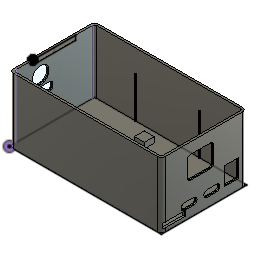
server_spiers_box v25 (Autodesk Fusion 360 design; units mm, degrees)
Autodesk Fusion 360 part; units mm, degrees
sketch "Base" plane through (0, 0, 0) normal (0, 1, 0) x (1, 0, 0) in component "Case"
  line L0 (0, 0) -> (107, 0)
  line L1 (107, 0) -> (107, 60)
  line L2 (107, 60) -> (0, 60)
  line L3 (0, 60) -> (0, 0)
  dimension "d6" = 107
  dimension "d7" = 60
  constraint horizontal L0
  constraint vertical L1
  constraint horizontal L2
  constraint vertical L3
  constraint coincident L0.start L3.end
  measures "d6" distance of L0.start L0.end
  measures "d7" distance of L0.start L2.end
extrude "Extrude1" add sketch "Base" along normal blind 46 makes body 1 in component "Case"
fillet "Fillet1" radius 3 4 edges at (107, 23, 0) (0, 23, 0) (107, 23, -60) (0, 23, -60) on bodies 1 in component "Case"
shell "Shell1" thickness 1.5 removed faces 1 at (36.6667, 46, -40) on bodies 1 in component "Case"
sketch "Knob" plane through (1.5, 0, 0) normal (1, 0, 0) x (0, 0, -1) in component "Case"
  line L0 (57, 46) -> (3, 46)
  line L1 (3, 1.5) -> (57, 1.5)
  line L2 (15, 46) -> (45, 46)
  line L3 (45, 46) -> (45, 43)
  line L4 (45, 43) -> (15, 43)
  line L5 (15, 43) -> (15, 46)
  line L6 (30, 46) -> (30, 43) construction
  line L7 (57, 1.5) -> (57, 46)
  line L8 (3, 46) -> (3, 1.5)
  dimension "d12" = 30
  dimension "d13" = 3
  constraint horizontal L2
  constraint vertical L3
  constraint horizontal L4
  constraint vertical L5
  constraint coincident L0 L2.start
  constraint midpoint L0 L6.start
  constraint midpoint L4 L6.end
  constraint vertical L6
  measures "d12" distance of L3.end L4.end
  measures "d13" distance of L2.end L3.end
extrude "Extrude2" add sketch "Knob" along normal blind 6 draft -45 contours L0 L2 L3 L4 L5 bodies 1 in component "Case"
ref_plane "WorkPlane2" through (53.5, 23, -30) normal (-1, 0, 0) x (0, 0, 1) in component "Case"
mirror "Mirror1" about plane through (53.5, 23, -30) normal (-1, 0, 0) of "Extrude2" in component "Case"
sketch "Top" plane through (0, 46, 0) normal (0, 1, 0) x (-1, 0, 0) in component "Top Cover"
  line L0 (-107, -3) -> (-107, -57)
  arc A0 (-107, -57) -> (-104, -60) centre (-104, -57) ccw
  line L1 (-104, -60) -> (-3, -60)
  arc A1 (-3, -60) -> (0, -57) centre (-3, -57) ccw
  line L2 (0, -57) -> (0, -3)
  arc A2 (0, -3) -> (-3, 0) centre (-3, -3) ccw
  line L3 (-3, 0) -> (-104, 0)
  arc A3 (-104, 0) -> (-107, -3) centre (-104, -3) ccw
  line L4 (-105.5, -15) -> (-105.5, -3)
  line L5 (-104, -1.5) -> (-3, -1.5)
  line L6 (-1.5, -3) -> (-1.5, -15)
  line L7 (-1.5, -15) -> (-1.5, -45)
  line L8 (-1.5, -45) -> (-1.5, -57)
  line L9 (-3, -58.5) -> (-104, -58.5)
  line L10 (-105.5, -45) -> (-105.5, -15)
  arc A4 (-104, -1.5) -> (-105.5, -3) centre (-104, -3) ccw
  arc A5 (-1.5, -3) -> (-3, -1.5) centre (-3, -3) ccw
  arc A6 (-3, -58.5) -> (-1.5, -57) centre (-3, -57) ccw
  arc A7 (-105.5, -57) -> (-104, -58.5) centre (-104, -57) ccw
  line L11 (-105.5, -57) -> (-105.5, -45)
extrude "Extrude1'" add sketch "Top" along normal blind 1.5 separate body contours L0 A0 L1 A1 L2 A2 L3 A3 | L4 L5 L6 L7 L8 L9 L10 A4 A5 A6 A7 L11 makes body 2 in component "Top Cover"
sketch "Lip" plane through (0, 46, 0) normal (0, -1, 0) x (1, 0, 0) in component "Top Cover"
  arc A0 (107, -3) -> (104, 0) centre (104, -3) ccw
  line L0 (104, 0) -> (3, 0)
  arc A1 (3, 0) -> (0, -3) centre (3, -3) ccw
  line L1 (0, -3) -> (0, -57)
  arc A2 (0, -57) -> (3, -60) centre (3, -57) ccw
  line L2 (3, -60) -> (104, -60)
  arc A3 (104, -60) -> (107, -57) centre (104, -57) ccw
  line L3 (107, -57) -> (107, -3)
  line L4 (107, -3) -> (107, -57)
  line L5 (105.3, -57) -> (105.3, -3)
  arc A4 (105.3, -3) -> (104, -1.7) centre (104, -3) ccw
  line L6 (104, -1.7) -> (3, -1.7)
  arc A5 (3, -1.7) -> (1.7, -3) centre (3, -3) ccw
  line L7 (1.7, -3) -> (1.7, -57)
  arc A6 (1.7, -57) -> (3, -58.3) centre (3, -57) ccw
  line L8 (3, -58.3) -> (104, -58.3)
  arc A7 (104, -58.3) -> (105.3, -57) centre (104, -57) ccw
  dimension "d19" = 1.7
  dimension "d31" = 1.7
  measures "d31" distance of L4 L5
extrude "Extrude2'" add sketch "Lip" along normal blind 3 contours L5 A4 L6 A5 L7 A6 L8 A7 bodies 2 in component "Top Cover"
extrude "Extrude3" cut sketch "Knob" along normal blind 3 draft -45 from surface at 0.2 contours L0 L2 L3 L4 L5 bodies 2 in component "Top Cover"
ref_plane "WorkPlane2" through (53.5, 0, 0) normal (1, 0, 0) x (0, 1, 0) in component "Top Cover"
mirror "Mirror1'" about plane through (53.5, 0, 0) normal (1, 0, 0) of "Extrude3" in component "Top Cover"
shell "Shell1'" thickness 1.5 removed faces 1 at (36.2333, 43, -25) on bodies 2 in component "Top Cover"
chamfer "Chamfer1" distance 0.6 angle 45 2 edges at (1.7, 43, -30) (105.3, 43, -30) on bodies 2 in component "Top Cover"
sketch "Esquisse1" plane through (107, 0, 0) normal (1, 0, 0) x (0, 0, -1)
  line L0 (57, 46) -> (3, 46)
  line L1 (3, 46) -> (3, 0)
  line L2 (3, 0) -> (57, 0)
  line L3 (57, 0) -> (57, 46)
  line L4 (38.75, 10.7) -> (32.25, 10.7)
  line L5 (32.25, 10.7) -> (32.25, 6.7)
  line L6 (32.25, 6.7) -> (38.75, 6.7)
  line L7 (38.75, 6.7) -> (38.75, 10.7)
  line L8 (38.75, 10.7) -> (32.25, 6.7) construction
  line L9 (32.25, 10.7) -> (38.75, 6.7) construction
  line L10 (60, 0) -> (60, 46)
  line L11 (0, 0) -> (60, 0)
  line L12 (22.75, 10.7) -> (16.25, 10.7)
  line L13 (16.25, 10.7) -> (16.25, 6.7)
  line L14 (16.25, 6.7) -> (22.75, 6.7)
  line L15 (22.75, 6.7) -> (22.75, 10.7)
  line L16 (22.75, 10.7) -> (16.25, 6.7) construction
  line L17 (16.25, 10.7) -> (22.75, 6.7) construction
  circle A0 centre (38.75, 8.7) radius 2
  circle A1 centre (32.25, 8.7) radius 2
  circle A2 centre (22.75, 8.7) radius 2
  circle A3 centre (16.25, 8.7) radius 2
  line L18 (34.5, 38) -> (20.5, 38)
  line L19 (18.5, 36) -> (18.5, 25)
  line L20 (20.5, 23) -> (34.5, 23)
  line L21 (36.5, 25) -> (36.5, 36)
  line L22 (36.5, 38) -> (18.5, 23) construction
  line L23 (18.5, 38) -> (36.5, 23) construction
  arc A4 (20.5, 38) -> (18.5, 36) centre (20.5, 36) ccw
  arc A5 (36.5, 36) -> (34.5, 38) centre (34.5, 36) ccw
  arc A6 (34.5, 23) -> (36.5, 25) centre (34.5, 25) ccw
  arc A7 (18.5, 25) -> (20.5, 23) centre (20.5, 25) ccw
  line L24 (54.25, 7.2) -> (44.75, 7.2)
  line L25 (44.75, 7.2) -> (44.75, 19.2)
  line L26 (44.75, 19.2) -> (54.25, 19.2)
  line L27 (54.25, 19.2) -> (54.25, 7.2)
  line L28 (54.25, 7.2) -> (44.75, 19.2) construction
  line L29 (44.75, 7.2) -> (54.25, 19.2) construction
  line L30 (0, 46) -> (0, 0)
  line L31 (16.5, 2.5) -> (1.5, 2.5)
  line L32 (1.5, 2.5) -> (1.5, 5.7)
  line L33 (1.5, 5.7) -> (16.5, 5.7)
  line L34 (16.5, 5.7) -> (16.5, 2.5)
  line L35 (16.5, 2.5) -> (1.5, 5.7) construction
  line L36 (1.5, 2.5) -> (16.5, 5.7) construction
  point P0 (35.5, 8.7)
  point P1 (19.5, 8.7)
  point P2 (27.5, 30.5)
  point P3 (49.5, 13.2)
  point P4 (9, 4.1)
  dimension "d36" = 6.5
  dimension "d37" = 4
  dimension "d39" = 8.7
  dimension "d40" = 6.5
  dimension "d41" = 4
  dimension "d42" = 16
  dimension "d43" = 8.7
  dimension "d44" = 4
  dimension "d45" = 4
  dimension "d46" = 4
  dimension "d47" = 4
  dimension "d69" = 18
  dimension "d70" = 15
  dimension "d71" = 30.5
  dimension "d72" = 32.5
  dimension "d82" = 2
  dimension "d83" = 2
  dimension "d84" = 2
  dimension "d85" = 2
  dimension "d233" = 9.5
  dimension "d234" = 12
  dimension "d235" = 13.2
  dimension "d236" = 10.5
  dimension "d237" = 14
  dimension "d260" = 15
  dimension "d261" = 3.2
  dimension "d262" = 9
  dimension "d335" = 4.6
  constraint horizontal L4
  constraint perpendicular L4 L5
  constraint parallel L4 L6
  constraint parallel L5 L7
  constraint coincident L8 P0
  constraint coincident L9 P0
  constraint horizontal L12
  constraint perpendicular L12 L13
  constraint parallel L12 L14
  constraint parallel L13 L15
  constraint coincident L16 P1
  constraint coincident L17 P1
  constraint coincident L4.start A0
  constraint midpoint L7 A0.centre
  constraint midpoint L5 A1.centre
  constraint midpoint L15 A2.centre
  constraint midpoint L13 A3.centre
  constraint horizontal L18
  constraint perpendicular L18 L19
  constraint parallel L18 L20
  constraint parallel L19 L21
  constraint coincident L22 P2
  constraint coincident L23 P2
  constraint coincident L23.start L18
  constraint coincident L23.start L19
  constraint tangent L18 A4
  constraint tangent L19 A4
  constraint coincident L22.start L18
  constraint coincident L22.start L21
  constraint tangent L18 A5
  constraint tangent L21 A5
  constraint coincident L23.end L20
  constraint coincident L23.end L21
  constraint tangent L20 A6
  constraint tangent L21 A6
  constraint coincident L22.end L19
  constraint coincident L22.end L20
  constraint tangent L19 A7
  constraint tangent L20 A7
  constraint horizontal L24
  constraint perpendicular L24 L25
  constraint parallel L24 L26
  constraint parallel L25 L27
  constraint coincident L28 P3
  constraint coincident L29 P3
  constraint horizontal L31
  constraint perpendicular L31 L32
  constraint parallel L31 L33
  constraint parallel L32 L34
  constraint coincident L35 P4
  constraint coincident L36 P4
  measures "d36" distance of L5.end L6.end
  measures "d37" distance of L4.end L5.end
  measures "d39" distance of P0 L11
  measures "d40" distance of L13.end L14.end
  measures "d41" distance of L12.end L13.end
  measures "d42" horizontal distance of P0 P1
  measures "d43" distance of L11 P1
  measures "d44" diameter of A0
  measures "d45" diameter of A1
  measures "d46" diameter of A2
  measures "d47" diameter of A3
  measures "d69" distance of L22.end L23.end
  measures "d70" distance of L23.start L22.end
  measures "d71" distance of L11 P2
  measures "d72" distance of L10 P2
  measures "d82" radius of A4
  measures "d83" radius of A5
  measures "d84" radius of A6
  measures "d85" radius of A7
  measures "d233" distance of L25.end L26.end
  measures "d234" distance of L24.end L25.end
  measures "d235" distance of L11 P3
  measures "d236" distance of L10 P3
  measures "d237" horizontal distance of P0 P3
  measures "d260" distance of L32.end L33.end
  measures "d261" distance of L31.end L32.end
  measures "d262" distance of L30 P4
  measures "d335" vertical distance of A3.centre P4
extrude "Extrusion3" cut sketch "Esquisse1" against normal blind 1.5 contours L4 L6 A0 A1 | L7 A0 | L7 A0 | L5 A1 | L5 A1 bodies 1 in component "Case"
extrude "Extrusion1" [suppressed]
extrude "Extrusion4" cut sketch "Esquisse1" against normal blind 1.5 contours L12 L14 A2 A3 | L15 A2 | L15 A2 | L13 A3 | L13 A3 bodies 1 in component "Case"
extrude "Extrusion9" cut sketch "Esquisse1" against normal blind 1.5 contours L18 L19 L20 L21 A4 A5 A6 A7 bodies 1 in component "Case"
fillet "Congé27" radius 0.375 8 edges at (105.5, 30.5, -18.5) (105.5, 23.5858, -19.0858) (105.5, 23, -27.5) (105.5, 23.5858, -35.9142) (105.5, 30.5, -36.5) (105.5, 37.4142, -35.9142) (105.5, 38, -27.5) (105.5, 37.4142, -19.0858) on bodies 1 in component "Case"
fillet "Congé28" radius 0.375 4 edges at (105.5, 6.7, -35.5) (105.5, 8.7, -40.75) (105.5, 10.7, -35.5) (105.5, 8.7, -30.25) on bodies 1 in component "Case"
fillet "Congé29" radius 0.375 4 edges at (105.5, 6.7, -19.5) (105.5, 8.7, -24.75) (105.5, 10.7, -19.5) (105.5, 8.7, -14.25) on bodies 1 in component "Case"
fillet "Congé30" radius 0.375 8 edges at (107, 30.5, -18.5) (107, 37.4142, -19.0858) (107, 38, -27.5) (107, 37.4142, -35.9142) (107, 30.5, -36.5) (107, 23.5858, -35.9142) (107, 23, -27.5) (107, 23.5858, -19.0858) on bodies 1 in component "Case"
fillet "Congé32" radius 0.375 4 edges at (107, 10.7, -19.5) (107, 8.7, -24.75) (107, 6.7, -19.5) (107, 8.7, -14.25) on bodies 1 in component "Case"
fillet "Congé33" radius 0.375 4 edges at (107, 10.7, -35.5) (107, 8.7, -40.75) (107, 6.7, -35.5) (107, 8.7, -30.25) on bodies 1 in component "Case"
extrude "Extrusion22" cut sketch "Esquisse1" against normal blind 1.5 contours L24 L25 L26 L27 bodies 1 in component "Case"
chamfer "Chanfrein6" distance 0.75 angle 45 1 edges at (105.5, 19.2, -49.5) on bodies 1 in component "Case"
fillet "Congé40" radius 0.375 3 edges at (105.5, 13.575, -44.75) (105.5, 7.2, -49.5) (105.5, 13.575, -54.25) on bodies 1 in component "Case"
fillet "Congé41" radius 0.375 4 edges at (107, 7.2, -49.5) (107, 13.2, -54.25) (107, 13.2, -44.75) (107, 19.2, -49.5) on bodies 1 in component "Case"
extrude "Extrusion29" cut sketch "Esquisse1" against normal blind 2.5 contours L1 L31 L33 L34 | L1 L31 L32 L33 bodies 1 in component "Case"
chamfer "Chanfrein9" distance 0.75 angle 45 2 edges at (105.5, 5.7, -9.75) (105.2247, 5.7, -2.134) on bodies 1 in component "Case"
fillet "Congé49" radius 0.375 1 edges at (107, 4.1, -16.5) on bodies 1 in component "Case"
fillet "Congé50" radius 0.375 2 edges at (106.8978, 5.7, -2.2235) (107, 5.7, -9.9375) on bodies 1 in component "Case"
sketch "Esquisse2" plane through (0, -0.0808, 0.0705) normal (-1, 0, 0) x (0, 0, 1)
  line L0 (-57.0705, 46.0808) -> (-57.0705, 0.0808)
  line L1 (-57.0705, 0.0808) -> (-3.0705, 0.0808)
  line L2 (-3.0705, 0.0808) -> (-3.0705, 46.0808)
  line L3 (-3.0705, 46.0808) -> (-57.0705, 46.0808)
  circle A0 centre (-20.5705, 34.0808) radius 5.5
  line L4 (-0.0705, 0.0808) -> (-0.0705, 46.0808)
  line L5 (-3.0705, 46.0808) -> (-57.0705, 46.0808)
  line L6 (-13.8705, 26.5808) -> (-27.2705, 26.5808)
  line L7 (-28.5705, 25.2808) -> (-28.5705, 22.8808)
  line L8 (-27.2705, 21.5808) -> (-13.8705, 21.5808)
  line L9 (-12.5705, 22.8808) -> (-12.5705, 25.2808)
  line L10 (-12.5705, 26.5808) -> (-28.5705, 21.5808) construction
  line L11 (-28.5705, 26.5808) -> (-12.5705, 21.5808) construction
  line L12 (-60.0705, 0.0808) -> (-0.0705, 0.0808)
  arc A1 (-27.2705, 26.5808) -> (-28.5705, 25.2808) centre (-27.2705, 25.2808) ccw
  arc A2 (-28.5705, 22.8808) -> (-27.2705, 21.5808) centre (-27.2705, 22.8808) ccw
  arc A3 (-12.5705, 25.2808) -> (-13.8705, 26.5808) centre (-13.8705, 25.2808) ccw
  arc A4 (-13.8705, 21.5808) -> (-12.5705, 22.8808) centre (-13.8705, 22.8808) ccw
  point P0 (-20.5705, 24.0808)
  dimension "d64" = 11
  dimension "d65" = 20.5
  dimension "d66" = 12
  dimension "d153" = 16
  dimension "d154" = 5
  dimension "d155" = 20.5
  dimension "d156" = 24
  dimension "d157" = 1.3
  dimension "d158" = 1.3
  dimension "d159" = 1.3
  dimension "d160" = 1.3
  constraint horizontal L6
  constraint perpendicular L6 L7
  constraint parallel L6 L8
  constraint parallel L7 L9
  constraint coincident L10 P0
  constraint coincident L11 P0
  constraint coincident L11.start L6
  constraint coincident L11.start L7
  constraint tangent L6 A1
  constraint tangent L7 A1
  constraint coincident L10.end L7
  constraint coincident L10.end L8
  constraint tangent L7 A2
  constraint tangent L8 A2
  constraint coincident L10.start L9
  constraint coincident L10.start L6
  constraint tangent L9 A3
  constraint tangent L6 A3
  constraint coincident L11.end L9
  constraint coincident L11.end L8
  constraint tangent L9 A4
  constraint tangent L8 A4
  measures "d64" diameter of A0
  measures "d65" distance of A0.centre L4
  measures "d66" distance of A0.centre L5
  measures "d153" distance of L10.end L11.end
  measures "d154" distance of L11.start L10.end
  measures "d155" distance of L4 P0
  measures "d156" distance of P0 L12
  measures "d157" radius of A1
  measures "d158" radius of A2
  measures "d159" radius of A3
  measures "d160" radius of A4
extrude "Extrusion6" cut sketch "Esquisse2" against normal blind 1.5 contours A0 bodies 1 in component "Case"
extrude "Extrusion20" cut sketch "Esquisse2" against normal blind 1.5 contours L6 L7 L8 L9 A1 A2 A3 A4 bodies 1 in component "Case"
fillet "Congé34" radius 0.375 1 edges at (0, 35.9889, -25.6278) on bodies 1 in component "Case"
fillet "Congé35" radius 0.375 8 edges at (0, 24, -28.5) (0, 26.1192, -28.1192) (0, 26.5, -20.5) (0, 26.1192, -12.8808) (0, 24, -12.5) (0, 21.8808, -12.8808) (0, 21.5, -20.5) (0, 21.8808, -28.1192) on bodies 1 in component "Case"
fillet "Congé36" radius 0.375 8 edges at (1.5, 24, -12.5) (1.5, 26.1192, -12.8808) (1.5, 26.5, -20.5) (1.5, 26.1192, -28.1192) (1.5, 24, -28.5) (1.5, 21.8808, -28.1192) (1.5, 21.5, -20.5) (1.5, 21.8808, -12.8808) on bodies 1 in component "Case"
fillet "Congé37" radius 0.375 1 edges at (1.5, 32.0111, -25.6278) on bodies 1 in component "Case"
sketch "Esquisse3" plane through (0, 1.5, 0) normal (0, 1, 0) x (-1, 0, 0)
  line L0 (-1.5, -57) -> (-1.5, -3)
  line L1 (-3, -1.5) -> (-104, -1.5)
  line L2 (-105.5, -3) -> (-105.5, -57)
  line L3 (-104, -58.5) -> (-3, -58.5)
  line L4 (-1.5, -38.5) -> (-5.5, -38.5)
  line L5 (-5.5, -38.5) -> (-5.5, -24.5)
  line L6 (-5.5, -24.5) -> (-1.5, -24.5)
  line L7 (-1.5, -24.5) -> (-1.5, -38.5)
  line L8 (-1.5, -38.5) -> (-5.5, -24.5) construction
  line L9 (-5.5, -38.5) -> (-1.5, -24.5) construction
  line L10 (0, -60) -> (0, 0)
  line L11 (0, 0) -> (-107, 0)
  line L12 (-91.5, -23.5) -> (-98.5, -23.5)
  line L13 (-98.5, -23.5) -> (-98.5, -16.5)
  line L14 (-98.5, -16.5) -> (-91.5, -16.5)
  line L15 (-91.5, -16.5) -> (-91.5, -23.5)
  line L16 (-91.5, -23.5) -> (-98.5, -16.5) construction
  line L17 (-98.5, -23.5) -> (-91.5, -16.5) construction
  line L18 (-107, 0) -> (-107, -60)
  line L19 (-107, -60) -> (0, -60)
  line L20 (-43.5, -15.5) -> (-50.5, -15.5)
  line L21 (-50.5, -15.5) -> (-50.5, -8.5)
  line L22 (-50.5, -8.5) -> (-43.5, -8.5)
  line L23 (-43.5, -8.5) -> (-43.5, -15.5)
  line L24 (-43.5, -15.5) -> (-50.5, -8.5) construction
  line L25 (-50.5, -15.5) -> (-43.5, -8.5) construction
  line L26 (-50.5, -44.5) -> (-43.5, -44.5)
  line L27 (-43.5, -44.5) -> (-43.5, -51.5)
  line L28 (-43.5, -51.5) -> (-50.5, -51.5)
  line L29 (-50.5, -51.5) -> (-50.5, -44.5)
  line L30 (-50.5, -44.5) -> (-43.5, -51.5) construction
  line L31 (-43.5, -44.5) -> (-50.5, -51.5) construction
  line L32 (-105.5, -51.5) -> (-98.5, -51.5)
  line L33 (-98.5, -51.5) -> (-98.5, -58.5)
  line L34 (-98.5, -58.5) -> (-105.5, -58.5)
  line L35 (-105.5, -58.5) -> (-105.5, -51.5)
  line L36 (-105.5, -51.5) -> (-98.5, -58.5) construction
  line L37 (-98.5, -51.5) -> (-105.5, -58.5) construction
  line L38 (-73.5, -3.5) -> (-77.5, -3.5)
  line L39 (-77.5, -3.5) -> (-77.5, -1.5)
  line L40 (-77.5, -1.5) -> (-73.5, -1.5)
  line L41 (-73.5, -1.5) -> (-73.5, -3.5)
  line L42 (-73.5, -3.5) -> (-77.5, -1.5) construction
  line L43 (-77.5, -3.5) -> (-73.5, -1.5) construction
  line L44 (-32.5, -3.5) -> (-28.5, -3.5)
  line L45 (-28.5, -3.5) -> (-28.5, -1.5)
  line L46 (-28.5, -1.5) -> (-32.5, -1.5)
  line L47 (-32.5, -1.5) -> (-32.5, -3.5)
  line L48 (-32.5, -3.5) -> (-28.5, -1.5) construction
  line L49 (-28.5, -3.5) -> (-32.5, -1.5) construction
  line L50 (-28.5, -1.5) -> (-32.5, -1.5)
  line L51 (-32.5, -3.5) -> (-28.5, -3.5)
  line L52 (-28.5, -3.5) -> (-28.5, -1.5)
  line L53 (-73.5, -3.5) -> (-77.5, -3.5)
  line L54 (-32.5, -1.5) -> (-32.5, -3.5)
  line L55 (-73.5, -1.5) -> (-73.5, -3.5)
  line L56 (-77.5, -1.5) -> (-73.5, -1.5)
  line L57 (-73.5, -3.5) -> (-77.5, -1.5) construction
  line L58 (-77.5, -3.5) -> (-73.5, -1.5) construction
  line L59 (-77.5, -3.5) -> (-77.5, -1.5)
  line L60 (-28.5, -3.5) -> (-32.5, -1.5) construction
  line L61 (-32.5, -3.5) -> (-28.5, -1.5) construction
  line L62 (-75, -58.5) -> (-76, -58.5)
  line L63 (-76, -58.5) -> (-76, -58)
  line L64 (-76, -58) -> (-75, -58)
  line L65 (-75, -58) -> (-75, -58.5)
  line L66 (-75, -58.5) -> (-76, -58) construction
  line L67 (-76, -58.5) -> (-75, -58) construction
  line L68 (-30, -58.5) -> (-31, -58.5)
  line L69 (-31, -58.5) -> (-31, -58)
  line L70 (-31, -58) -> (-30, -58)
  line L71 (-30, -58) -> (-30, -58.5)
  line L72 (-30, -58.5) -> (-31, -58) construction
  line L73 (-31, -58.5) -> (-30, -58) construction
  arc A0 (-3, -58.5) -> (-1.5, -57) centre (-3, -57) ccw
  arc A1 (-1.5, -3) -> (-3, -1.5) centre (-3, -3) ccw
  arc A2 (-104, -1.5) -> (-105.5, -3) centre (-104, -3) ccw
  line L74 (-1.5, -30.5) -> (-2, -30.5)
  line L75 (-2, -30.5) -> (-2, -32.5)
  line L76 (-2, -32.5) -> (-1.5, -32.5)
  line L77 (-1.5, -32.5) -> (-1.5, -30.5)
  line L78 (-1.5, -30.5) -> (-2, -32.5) construction
  line L79 (-2, -30.5) -> (-1.5, -32.5) construction
  point P0 (-3.5, -31.5)
  point P1 (-95, -20)
  point P2 (-47, -12)
  point P3 (-47, -48)
  point P4 (-102, -55)
  point P5 (-75.5, -2.5)
  point P6 (-30.5, -2.5)
  point P7 (-75.5, -2.5)
  point P8 (-30.5, -2.5)
  point P9 (-75.5, -58.25)
  point P10 (-30.5, -58.25)
  point P11 (-1.75, -31.5)
  dimension "d86" = 4
  dimension "d87" = 14
  dimension "d92" = 3.5
  dimension "d93" = 31.5
  dimension "d96" = 7
  dimension "d97" = 7
  dimension "d98" = 12
  dimension "d99" = 20
  dimension "d104" = 7
  dimension "d105" = 7
  dimension "d106" = 12
  dimension "d107" = 60
  dimension "d108" = 7
  dimension "d109" = 7
  dimension "d110" = 12
  dimension "d111" = 60
  dimension "d253" = 7
  dimension "d254" = 7
  dimension "d255" = 5
  dimension "d256" = 5
  dimension "d271" = 4
  dimension "d272" = 2
  dimension "d273" = 1
  dimension "d274" = 30
  dimension "d275" = 4
  dimension "d276" = 2
  dimension "d277" = 1
  dimension "d278" = 75
  dimension "d279" = 4
  dimension "d280" = 2
  dimension "d281" = 4
  dimension "d282" = 2
  dimension "d283" = 1
  dimension "d284" = 0.5
  dimension "d285" = 0.25
  dimension "d286" = 30
  dimension "d287" = 1
  dimension "d288" = 0.5
  dimension "d289" = 0.25
  dimension "d290" = 75
  dimension "d326" = 0.5
  dimension "d327" = 2
  dimension "d328" = 0.25
  constraint horizontal L4
  constraint perpendicular L4 L5
  constraint parallel L4 L6
  constraint parallel L5 L7
  constraint coincident L8 P0
  constraint coincident L9 P0
  constraint horizontal L12
  constraint perpendicular L12 L13
  constraint parallel L12 L14
  constraint parallel L13 L15
  constraint coincident L16 P1
  constraint coincident L17 P1
  constraint horizontal L20
  constraint perpendicular L20 L21
  constraint parallel L20 L22
  constraint parallel L21 L23
  constraint coincident L24 P2
  constraint coincident L25 P2
  constraint horizontal L26
  constraint perpendicular L26 L27
  constraint parallel L26 L28
  constraint parallel L27 L29
  constraint coincident L30 P3
  constraint coincident L31 P3
  constraint horizontal L32
  constraint perpendicular L32 L33
  constraint parallel L32 L34
  constraint parallel L33 L35
  constraint coincident L36 P4
  constraint coincident L37 P4
  constraint horizontal L38
  constraint perpendicular L38 L39
  constraint parallel L38 L40
  constraint parallel L39 L41
  constraint coincident L42 P7
  constraint coincident L43 P7
  constraint horizontal L44
  constraint perpendicular L44 L45
  constraint parallel L44 L46
  constraint parallel L45 L47
  constraint coincident L48 P8
  constraint coincident L49 P8
  constraint horizontal L53
  constraint perpendicular L53 L59
  constraint parallel L53 L56
  constraint parallel L55 L59
  constraint coincident P7 L57
  constraint coincident P7 L58
  constraint horizontal L51
  constraint perpendicular L51 L52
  constraint parallel L50 L51
  constraint parallel L52 L54
  constraint coincident P8 L61
  constraint coincident P8 L60
  constraint horizontal L62
  constraint perpendicular L62 L63
  constraint parallel L62 L64
  constraint parallel L63 L65
  constraint coincident L66 P9
  constraint coincident L67 P9
  constraint horizontal L68
  constraint perpendicular L68 L69
  constraint parallel L68 L70
  constraint parallel L69 L71
  constraint coincident L72 P10
  constraint coincident L73 P10
  constraint horizontal L74
  constraint perpendicular L74 L75
  constraint parallel L74 L76
  constraint parallel L75 L77
  constraint coincident L78 P11
  constraint coincident L79 P11
  measures "d86" distance of L5.end L6.end
  measures "d87" distance of L4.end L5.end
  measures "d92" distance of P0 L10
  measures "d93" distance of P0 L11
  measures "d96" distance of L13.end L14.end
  measures "d97" distance of L12.end L13.end
  measures "d98" distance of P1 L18
  measures "d99" distance of L11 P1
  measures "d104" distance of L21.end L22.end
  measures "d105" distance of L20.end L21.end
  measures "d106" distance of L11 P2
  measures "d107" distance of L18 P2
  measures "d108" distance of L27.end L28.end
  measures "d109" distance of L26.end L27.end
  measures "d110" distance of L19 P3
  measures "d111" distance of L18 P3
  measures "d253" distance of L33.end L34.end
  measures "d254" distance of L32.end L33.end
  measures "d255" distance of L19 P4
  measures "d256" distance of L18 P4
  measures "d271" distance of L39.end L40.end
  measures "d272" distance of L38.end L39.end
  measures "d273" distance of L1 P7
  measures "d274" distance of L2 P7
  measures "d275" distance of L45.end L46.end
  measures "d276" distance of L44.end L45.end
  measures "d277" distance of L1 P8
  measures "d278" distance of L2 P8
  measures "d279" distance of L39.end L40.end
  measures "d280" distance of L38.end L39.end
  measures "d281" distance of L46.end L45.end
  measures "d282" distance of L45.end L44.end
  measures "d283" distance of L63.end L64.end
  measures "d284" distance of L62.end L63.end
  measures "d285" distance of L3 P9
  measures "d286" distance of L2 P9
  measures "d287" distance of L69.end L70.end
  measures "d288" distance of L68.end L69.end
  measures "d289" distance of L3 P10
  measures "d290" distance of L2 P10
  measures "d326" distance of L75.end L76.end
  measures "d327" distance of L74.end L75.end
  measures "d328" distance of L0 P11
extrude "Extrusion24" add sketch "Esquisse3" along normal blind 29 contours L1 L38 L39 L40 L41 L53 L55 L56 L59 bodies 1 in component "Case"
extrude "Extrusion25" add sketch "Esquisse3" along normal blind 29 contours L1 L44 L45 L46 L47 L50 L51 L52 L54 bodies 1 in component "Case"
extrude "Extrusion26" add sketch "Esquisse3" along normal blind 29 contours L3 L68 L69 L70 L71 | L3 L62 L63 L64 L65 bodies 1 in component "Case"
extrude "Extrusion10" add sketch "Esquisse3" along normal blind 4 contours L0 L4 L5 L6 L7 L74 L75 L76 | L0 L7 L74 L75 L76 L77 bodies 1 in component "Case"
extrude "Extrusion30" add sketch "Esquisse3" along normal blind 4 contours L12 L13 L14 L15 | L20 L21 L22 L23 | L26 L27 L28 L29 bodies 1 in component "Case"
extrude "Extrusion5" add sketch "Esquisse3" along normal blind 12 separate body contours L0 L7 L74 L75 L76 L77 makes body 3
chamfer "Chanfrein1" distance 0.5 distance2 5 1 edges at (2, 13.5, -31.5) measured on face at (1.6667, 13.5, -31.8333) on bodies 3
chamfer "Chanfrein10" distance 2 distance2 7 2 edges at (30.5, 30.5, -3.5) (75.5, 30.5, -3.5) measured on face at (31.1667, 30.5, -2.1667) measured on face at (76.1667, 30.5, -2.8333) on bodies 1 in component "Case"
component "Enclosure" placed x (1, 0, 0) y (0, 1, 0) z (0, 0, 1) at (0, 0, 0)
component "Case" placed x (1, 0, 0) y (0, 1, 0) z (0, 0, 1) at (0, 0, 0) in component "Enclosure"
component "Top Cover" placed x (1, 0, 0) y (0, 1, 0) z (0, 0, 1) at (0, 0, 0) in component "Enclosure"
equation "Width = Width_internal + ( 2 * shell )"
equation "length = Length_internal + ( 2 * shell )"
equation "heigth = 42 mm + support_ep"
equation "shell = 1.5 mm"
equation "gap = 0.2 mm"
equation "d6 = length"
equation "d7 = Width"
equation "d8 = heigth"
equation "d10 = shell * 2"
equation "d11 = shell"
equation "d12 = Width / 2"
equation "d13 = shell * 2"
equation "d17 = shell"
equation "d19 = shell + gap"
equation "d20 = shell * 2"
equation "d23 = shell * 2"
equation "d26 = shell"
equation "d31 = shell + gap"
equation "d33 = length / 2"
equation "Width_internal = 57 mm"
equation "Length_internal = 104 mm"
equation "d39 = 3.2 mm + support_ep + shell"
equation "d43 = 3.2 mm + support_ep + shell"
equation "d51 = -shell"
equation "d53 = -shell"
equation "d55 = -shell"
equation "d65 = d155"
equation "d67 = -shell"
equation "d71 = 8 mm + 21 mm + shell"
equation "d72 = 9 mm + 22 mm + shell"
equation "d80 = -shell"
equation "d87 = support_coté * 2"
equation "d88 = support_ep"
equation "support_coté = 7 mm"
equation "support_ep = 4 mm"
equation "d92 = d86 / 2 + shell"
equation "d93 = Width / 2 + shell"
equation "d96 = support_coté"
equation "d97 = support_coté"
equation "d98 = 7 mm + support_coté / 2 + shell"
equation "d99 = 15 mm + support_coté / 2 + shell"
equation "d104 = support_coté"
equation "d105 = support_coté"
equation "d106 = support_coté / 2 + shell + 7 mm"
equation "d107 = support_coté / 2 + shell + 55 mm"
equation "d108 = support_coté"
equation "d109 = support_coté"
equation "d110 = support_coté / 2 + shell + 7 mm"
equation "d111 = support_coté / 2 + shell + 55 mm"
equation "d155 = 19 mm + shell"
equation "d156 = 18.5 mm + support_ep + shell"
equation "d208 = shell / 4"
equation "d210 = shell / 4"
equation "d212 = shell / 4"
equation "d214 = shell / 4"
equation "d218 = shell / 4"
equation "d220 = shell / 4"
equation "d221 = -shell"
equation "d224 = shell / 4"
equation "d226 = shell / 4"
equation "d228 = shell / 4"
equation "d232 = shell / 4"
equation "d235 = 7.7 mm + support_ep + shell"
equation "d236 = 9 mm + shell"
equation "d246 = -shell"
equation "d248 = shell / 2"
equation "d250 = shell / 4"
equation "d252 = shell / 4"
equation "d255 = d254 / 2 + shell"
equation "d256 = support_coté / 2 + shell"
equation "d262 = d260 / 2 + shell"
equation "cale_coté_alim = 0.5 mm"
equation "cale_coté_usb = 2 mm"
equation "cale_hauteur = support_ep + 25 mm"
equation "d271 = 2 * cale_coté_usb"
equation "d272 = cale_coté_usb"
equation "d273 = cale_coté_usb / 2"
equation "d275 = 2 * cale_coté_usb"
equation "d276 = cale_coté_usb"
equation "d277 = cale_coté_usb / 2"
equation "d279 = 2 * cale_coté_usb"
equation "d280 = cale_coté_usb"
equation "d281 = 2 * cale_coté_usb"
equation "d282 = cale_coté_usb"
equation "d283 = 2 * cale_coté_alim"
equation "d284 = cale_coté_alim"
equation "d285 = cale_coté_alim / 2"
equation "d287 = 2 * cale_coté_alim"
equation "d288 = cale_coté_alim"
equation "d289 = cale_coté_alim / 2"
equation "d291 = cale_hauteur"
equation "d293 = cale_hauteur"
equation "d295 = cale_hauteur"
equation "d310 = -shell - 1 mm"
equation "d316 = support_ep"
equation "d319 = shell / 2"
equation "d321 = shell / 4"
equation "d323 = shell / 4"
equation "d328 = d326 / 2"
equation "d329 = support_ep + 3 mm + 5 mm"
equation "d331 = d326"
equation "d332 = d329 - support_ep - 3 mm"
equation "d333 = cale_coté_usb"
equation "d335 = 1 mm + d41 / 2 + d261 / 2"
